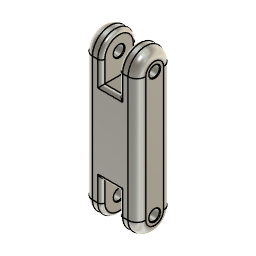
hand_montage v0 (Autodesk Fusion 360 archive; units mm, degrees)
design "proximal v1"
Autodesk Fusion 360 part; units mm, degrees
sketch "Çizim1" plane through (0, 0, 0) normal (0, 1, 0) x (1, 0, 0)
  line L0 (-15, 45) -> (15, 45)
  line L1 (15, 45) -> (15, -45)
  line L2 (15, -45) -> (-15, -45)
  line L3 (-15, -45) -> (-15, 45)
  line L4 (-15, 45) -> (15, -45) construction
  line L5 (15, 45) -> (-15, -45) construction
  dimension "d1" = 30
  dimension "d2" = 90
  constraint horizontal L0
  constraint perpendicular L0 L1
  constraint parallel L0 L2
  constraint parallel L1 L3
  constraint coincident L4 origin
  constraint coincident L5 origin
  measures "d1" distance of L1.end L2.end
  measures "d2" distance of L0.end L1.end
extrude "Ekstrüzyon1" add sketch "Çizim1" along normal blind 20
sketch "Çizim2" plane through (0, 0, 0) normal (0, -1, 0) x (1, 0, 0)
  line L0 (15, 45) -> (-15, 45)
  line L1 (-15, 45) -> (-15, -45)
  line L2 (-15, -45) -> (15, -45)
  line L3 (15, -45) -> (15, 45)
  line L4 (-5, 67) -> (5, 67)
  line L5 (5, 67) -> (5, 23)
  line L6 (5, 23) -> (-5, 23)
  line L7 (-5, 23) -> (-5, 67)
  line L8 (-5, 67) -> (5, 23) construction
  line L9 (5, 67) -> (-5, 23) construction
  point P0 (0, 45)
  dimension "d5" = 10
  dimension "d6" = 44
  constraint horizontal L4
  constraint perpendicular L4 L5
  constraint parallel L4 L6
  constraint parallel L5 L7
  constraint coincident L8 P0
  constraint coincident L9 P0
  constraint midpoint L0 P0
  measures "d5" distance of L5.end L6.end
  measures "d6" distance of L4.end L5.end
extrude "Ekstrüzyon2" cut sketch "Çizim2" against normal blind 70 contours L0 L5 L6 L7
sketch "Çizim3" plane through (0, 0, 0) normal (0, -1, 0) x (1, 0, 0)
  line L0 (-5, 23) -> (-5, 45)
  line L1 (-5, 45) -> (-15, 45)
  line L2 (-15, 45) -> (-15, -45)
  line L3 (-15, -45) -> (15, -45)
  line L4 (15, -45) -> (15, 45)
  line L5 (15, 45) -> (5, 45)
  line L6 (5, 45) -> (5, 23)
  line L7 (5, 23) -> (-5, 23)
  line L8 (-5, -23) -> (5, -23)
  line L9 (5, -23) -> (5, -67)
  line L10 (5, -67) -> (-5, -67)
  line L11 (-5, -67) -> (-5, -23)
  line L12 (-5, -23) -> (5, -67) construction
  line L13 (5, -23) -> (-5, -67) construction
  point P0 (0, -45)
  dimension "d9" = 10
  dimension "d10" = 44
  constraint horizontal L8
  constraint perpendicular L8 L9
  constraint parallel L8 L10
  constraint parallel L9 L11
  constraint coincident L12 P0
  constraint coincident L13 P0
  constraint midpoint L3 P0
  measures "d9" distance of L9.end L10.end
  measures "d10" distance of L8.end L9.end
extrude "Ekstrüzyon3" cut sketch "Çizim3" against normal blind 210 contours L3 L8 L9 L11
sketch "Çizim4" plane through (15, 0, 0) normal (1, 0, 0) x (0, 1, 0)
  line L0 (0, 45) -> (0, -45)
  line L1 (0, -45) -> (20, -45)
  line L2 (20, -45) -> (20, 45)
  line L3 (20, 45) -> (0, 45)
  circle A0 centre (10, 35) radius 10
  circle A1 centre (10, -35) radius 10
  circle A2 centre (10, 35) radius 3
  circle A3 centre (10, -35) radius 3
  dimension "d13" = 20
  dimension "d14" = 20
  dimension "d15" = 6
  dimension "d16" = 6
  constraint concentric A0 A2
  constraint concentric A1 A3
  measures "d13" diameter of A0
  measures "d14" diameter of A1
  measures "d15" diameter of A2
  measures "d16" diameter of A3
extrude "Ekstrüzyon4" cut sketch "Çizim4" against normal blind 52 contours A2 | A3
extrude "Ekstrüzyon5" cut sketch "Çizim4" against normal blind 115 contours L0 L3 A0 | L2 L3 A0 | L0 L1 A1 | L1 L2 A1
fillet "Radyus1" radius 2 16 edges at (-5, 20, 29) (-5, 10, 45) (-5, 0, 29) (5, 0, 29) (5, 10, 45) (5, 20, 29) (5, 0, -29) (5, 10, -45) (5, 20, -29) (-5, 20, -29) (-5, 10, -45) (-5, 0, -29) (0, 0, -23) (0, 0, 23) (0, 20, 23) (0, 20, -23)
fillet "Radyus2" radius 5 8 edges at (15, 10, 45) (15, 20, 0) (15, 10, -45) (15, 0, 0) (-15, 10, -45) (-15, 20, 0) (-15, 10, 45) (-15, 0, 0)
fillet "Radyus3" radius 0.3 8 edges at (-5, 7.203, 36.0848) (-15, 7.203, 33.9152) (5, 7.203, 33.9152) (15, 7.203, 36.0848) (15, 7.203, -33.9152) (5, 7.203, -36.0848) (-5, 7.203, -33.9152) (-15, 7.203, -36.0848)

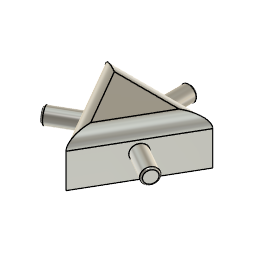
design "wrist_integrator"
Autodesk Fusion 360 part; units mm, degrees
sketch "Çizim5" plane through (0, 0, 0) normal (0, 0, 1) x (1, 0, 0)
  line L0 (-34.641, 20) -> (0, -40)
  line L1 (0, -40) -> (34.641, 20)
  line L2 (34.641, 20) -> (-34.641, 20)
  dimension "d17" = 20
  measures "d17" distance of origin L2
extrude "Ekstrüzyon5" add sketch "Çizim5" along normal blind 30
sketch "Çizim6" plane through (17.3205, -10, 0) normal (0.866025, -0.5, 0) x (0.5, 0.866025, 0)
  line L0 (-34.641, 0) -> (34.641, 0)
  line L1 (34.641, 0) -> (34.641, 30)
  line L2 (34.641, 30) -> (-34.641, 30)
  line L3 (-34.641, 30) -> (-34.641, 0)
  circle A0 centre (0, 15) radius 5
  dimension "d20" = 10
  measures "d20" diameter of A0
extrude "Ekstrüzyon6" add sketch "Çizim6" along normal blind 20 contours A0
sketch "Çizim7" plane through (0, 20, 0) normal (0, 1, 0) x (-1, 0, 0)
  line L0 (-34.641, 0) -> (34.641, 0)
  line L1 (34.641, 0) -> (34.641, 30)
  line L2 (34.641, 30) -> (-34.641, 30)
  line L3 (-34.641, 30) -> (-34.641, 0)
  circle A0 centre (0, 15) radius 5
  dimension "d23" = 10
  measures "d23" diameter of A0
extrude "Ekstrüzyon7" add sketch "Çizim7" along normal blind 20 contours A0
sketch "Çizim8" plane through (-17.3205, -10, 0) normal (-0.866025, -0.5, 0) x (0.5, -0.866025, 0)
  line L0 (-34.641, 0) -> (34.641, 0)
  line L1 (34.641, 0) -> (34.641, 30)
  line L2 (34.641, 30) -> (-34.641, 30)
  line L3 (-34.641, 30) -> (-34.641, 0)
  circle A0 centre (0, 15) radius 5
  dimension "d26" = 10
  measures "d26" diameter of A0
extrude "Ekstrüzyon8" add sketch "Çizim8" along normal blind 20 contours A0
fillet "Radyus3" radius 8 3 edges at (-17.3205, -10, 30) (0, 20, 30) (17.3205, -10, 30)
fillet "Radyus4" radius 1 3 edges at (32.3102, -24.0371, 13.1919) (4.6616, 40, 13.1919) (-36.9718, -15.9629, 13.1919)

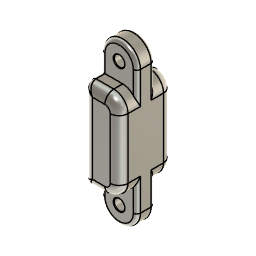
design "middle v1"
Autodesk Fusion 360 part; units mm, degrees
sketch "Çizim1" plane through (0, 0, 0) normal (0, 1, 0) x (1, 0, 0)
  circle A0 centre (0, 0) radius 10
  dimension "d1" = 20
  constraint coincident A0.centre origin
  measures "d1" diameter of A0
extrude "Ekstrüzyon1" add sketch "Çizim1" along normal blind 10
sketch "Çizim2" plane through (0, 0, 0) normal (0, -1, 0) x (1, 0, 0)
  circle A0 centre (0, 0) radius 10
  line L0 (-10, 0) -> (10, 0)
  line L1 (10, 0) -> (10, -80)
  line L2 (10, -80) -> (-10, -80)
  line L3 (-10, -80) -> (-10, 0)
  dimension "d4" = 80
  constraint horizontal L0
  constraint vertical L1
  constraint horizontal L2
  constraint vertical L3
  constraint coincident A0 L0.start
  measures "d4" distance of L0.start L2.end
extrude "Ekstrüzyon2" add sketch "Çizim2" against normal blind 10 contours A0 L1 L2 L3
sketch "Çizim3" plane through (0, 0, 0) normal (0, -1, 0) x (1, 0, 0)
  arc A0 (10, 0) -> (-10, 0) centre (0, 0) ccw
  line L0 (-10, 0) -> (-10, -80)
  line L1 (-10, -80) -> (10, -80)
  line L2 (10, -80) -> (10, 0)
  line L3 (-10, -10) -> (10, -10)
  line L4 (10, -10) -> (10, -60)
  line L5 (10, -60) -> (-10, -60)
  line L6 (-10, -60) -> (-10, -10)
  dimension "d7" = 20
  dimension "d8" = 50
  constraint horizontal L3
  constraint vertical L4
  constraint horizontal L5
  constraint vertical L6
  constraint coincident L0 L3.start
  measures "d7" distance of L3.start L3.end
  measures "d8" distance of L3.start L5.end
extrude "Ekstrüzyon3" add sketch "Çizim3" along normal blind 10 contours L0 L2 L3 L4 L5 L6
sketch "Çizim4" plane through (0, 10, 0) normal (0, 1, 0) x (-1, 0, 0)
  arc A0 (10, 0) -> (-10, 0) centre (0, 0) ccw
  line L0 (-10, 0) -> (-10, -80)
  line L1 (-10, -80) -> (10, -80)
  line L2 (10, -80) -> (10, 0)
  line L3 (-10, -10) -> (10, -10)
  line L4 (10, -10) -> (10, -60)
  line L5 (10, -60) -> (-10, -60)
  line L6 (-10, -60) -> (-10, -10)
  dimension "d11" = 50
  constraint horizontal L3
  constraint vertical L4
  constraint horizontal L5
  constraint vertical L6
  constraint coincident L0 L3.start
  measures "d11" distance of L3.start L5.end
extrude "Ekstrüzyon4" add sketch "Çizim4" along normal blind 10 contours L0 L2 L3 L4 L5 L6
sketch "Çizim5" plane through (0, 0, 0) normal (0, -1, 0) x (1, 0, 0)
  line L0 (10, -60) -> (-10, -60)
  line L1 (-10, -60) -> (-10, -80)
  line L2 (-10, -80) -> (10, -80)
  line L3 (10, -80) -> (10, -60)
  circle A0 centre (0, -70) radius 10
  dimension "d14" = 20
  measures "d14" diameter of A0
extrude "Ekstrüzyon5" cut sketch "Çizim5" against normal blind 15 contours L2 L3 A0 | L1 L2 A0
sketch "Çizim6" plane through (0, 10, 0) normal (0, 1, 0) x (-1, 0, 0)
  line L0 (-10, -10) -> (10, -10)
  line L1 (10, -10) -> (10, 0)
  arc A0 (10, 0) -> (-10, 0) centre (0, 0) ccw
  line L2 (-10, 0) -> (-10, -10)
  circle A1 centre (0, 0) radius 3
  dimension "d17" = 6
  constraint coincident A0.centre A1.centre
  measures "d17" diameter of A1
extrude "Ekstrüzyon6" cut sketch "Çizim6" against normal blind 105 contours A1
sketch "Çizim7" plane through (0, 10, 0) normal (0, 1, 0) x (-1, 0, 0)
  arc A0 (-10, -70) -> (10, -70) centre (0, -70) ccw
  line L0 (10, -70) -> (10, -60)
  line L1 (10, -60) -> (-10, -60)
  line L2 (-10, -60) -> (-10, -70)
  circle A1 centre (0, -70) radius 3
  dimension "d20" = 6
  constraint concentric A0 A1
  measures "d20" diameter of A1
extrude "Ekstrüzyon7" cut sketch "Çizim7" against normal blind 34 contours A1
fillet "Radyus1" radius 2 12 edges at (-10, 0, -5) (0, 0, 10) (10, 0, -5) (-10, 10, -5) (0, 10, 10) (10, 10, -5) (10, 0, -65) (0, 0, -80) (-10, 0, -65) (10, 10, -65) (0, 10, -80) (-10, 10, -65)
fillet "Radyus2" radius 5 2 faces at (-3.3333, -10, -43.3333) (3.3333, 20, -43.3333)
fillet "Radyus3" radius 0.3 4 edges at (2.797, 0, -1.0848) (2.797, 10, 1.0848) (2.797, 0, -71.0848) (2.797, 10, -68.9152)
fillet "Radyus4" radius 8 8 edges at (10, -1.5, -10) (8.5355, -8.5355, -11.4645) (10, 11.5, -10) (8.5355, 18.5355, -11.4645) (10, -1.5, -60) (8.5355, -8.5355, -58.5355) (10, 11.5, -60) (8.5355, 18.5355, -58.5355)
fillet "Radyus5" radius 2 8 edges at (-10, 11.5, -10) (-8.5355, 18.5355, -11.4645) (-10, -1.5, -10) (-8.5355, -8.5355, -11.4645) (-10, 11.5, -60) (-8.5355, 18.5355, -58.5355) (-10, -1.5, -60) (-8.5355, -8.5355, -58.5355)

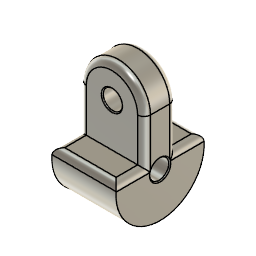
design "knuckle"
Autodesk Fusion 360 part; units mm, degrees
sketch "Çizim1" plane through (0, 0, 0) normal (0, 1, 0) x (1, 0, 0)
  circle A0 centre (0, 0) radius 10
  dimension "d1" = 20
  constraint coincident A0.centre origin
  measures "d1" diameter of A0
extrude "Ekstrüzyon1" add sketch "Çizim1" along normal blind 10
sketch "Çizim2" plane through (0, 0, 0) normal (0, -1, 0) x (1, 0, 0)
  circle A0 centre (0, 0) radius 10
  line L0 (-10, 0) -> (10, 0)
  line L1 (10, 0) -> (10, -30)
  line L2 (10, -30) -> (-10, -30)
  line L3 (-10, -30) -> (-10, 0)
  dimension "d4" = 30
  constraint horizontal L0
  constraint vertical L1
  constraint horizontal L2
  constraint vertical L3
  constraint coincident A0 L0.start
  measures "d4" distance of L0.start L2.end
extrude "Ekstrüzyon2" add sketch "Çizim2" against normal blind 10 contours A0 L1 L2 L3
sketch "Çizim3" plane through (10, 0, 0) normal (1, 0, 0) x (0, 1, 0)
  line L0 (0, 0) -> (0, -30)
  line L1 (0, -30) -> (10, -30)
  line L2 (10, -30) -> (10, 0)
  line L3 (10, 0) -> (0, 0)
  circle A0 centre (5, -16.25) radius 13.75
  dimension "d7" = 27.5
  measures "d7" diameter of A0
extrude "Ekstrüzyon3" add sketch "Çizim3" against normal blind 20 contours L0 A0 | L2 A0
sketch "Çizim4" plane through (10, 0, 0) normal (1, 0, 0) x (0, 1, 0)
  line L0 (0, 0) -> (0, -3.4413)
  arc A0 (0, -3.4413) -> (0, -29.0587) centre (5, -16.25) ccw
  line L1 (0, -29.0587) -> (0, -30)
  line L2 (0, -30) -> (10, -30)
  line L3 (10, -30) -> (10, -29.0587)
  arc A1 (10, -29.0587) -> (10, -3.4413) centre (5, -16.25) ccw
  line L4 (10, -3.4413) -> (10, 0)
  line L5 (10, 0) -> (0, 0)
  circle A2 centre (5, -16.25) radius 13.75
  constraint tangent A1 A2
extrude "Ekstrüzyon4" cut sketch "Çizim4" against normal blind 35 contours L1 L2 A2 | L2 L3 A2
sketch "Çizim5" plane through (0, 0, 0) normal (0, -1, 0) x (1, 0, 0)
  line L0 (-10, -3.4413) -> (10, -3.4413)
  line L1 (10, -3.4413) -> (10, 0)
  arc A0 (10, 0) -> (-10, 0) centre (0, 0) ccw
  line L2 (-10, 0) -> (-10, -3.4413)
  circle A1 centre (0, 0) radius 3
  dimension "d12" = 6
  constraint coincident A0.centre A1.centre
  measures "d12" diameter of A1
extrude "Ekstrüzyon5" cut sketch "Çizim5" against normal blind 80 contours A1
sketch "Çizim6" plane through (10, 0, 0) normal (1, 0, 0) x (0, 1, 0)
  arc A0 (0, -3.4413) -> (10, -3.4413) centre (5, -16.25) ccw
  line L0 (10, -3.4413) -> (10, 0)
  line L1 (10, 0) -> (0, 0)
  line L2 (0, 0) -> (0, -3.4413)
  line L3 (0, -3.4413) -> (10, -3.4413)
  line L4 (10, -3.4413) -> (10, -13.4413)
  line L5 (10, -13.4413) -> (0, -13.4413)
  line L6 (0, -13.4413) -> (0, -3.4413)
  line L7 (-8.4601, -13.4413) -> (18.4601, -13.4413)
  dimension "d15" = 10
  constraint horizontal L3
  constraint vertical L4
  constraint horizontal L5
  constraint vertical L6
  constraint coincident A0.start L2.end
  constraint coincident A0 L7.start
  constraint coincident A0 L7.end
  constraint perpendicular L6 L7
  measures "d15" distance of A0.start L5.end
extrude "Ekstrüzyon6" cut sketch "Çizim6" against normal blind 39 contours A0 L6 L7 | A0 L4 L7
fillet "Radyus1" radius 2 6 edges at (0, 18.4601, -13.4413) (0, -8.4601, -13.4413) (10, -4.23, -13.4413) (10, 14.23, -13.4413) (-10, -4.23, -13.4413) (-10, 14.23, -13.4413)
fillet "Radyus2" radius 2 6 edges at (-10, 10, -7.7207) (0, 10, 10) (10, 10, -7.7207) (-10, 0, -7.7207) (0, 0, 10) (10, 0, -7.7207)
fillet "Radyus3" radius 0.3 1 edges at (-2.797, 10, -1.0848)
sketch "Çizim7" plane through (10, 0, 0) normal (1, 0, 0) x (0, 1, 0)
  line L0 (2, -15.4413) -> (-8.7262, -15.4413)
  arc A0 (-8.7262, -15.4413) -> (18.7262, -15.4413) centre (5, -16.25) ccw
  line L1 (18.7262, -15.4413) -> (8, -15.4413)
  line L2 (8, -15.4413) -> (8, 0)
  line L3 (8, 0) -> (2, 0)
  line L4 (2, 0) -> (2, -15.4413)
  circle A1 centre (5, -16.25) radius 13.75
  circle A2 centre (5, -16.25) radius 3
  dimension "d24" = 27.5
  dimension "d25" = 6
  constraint concentric A1 A2
  measures "d24" diameter of A1
  measures "d25" diameter of A2
extrude "Ekstrüzyon7" cut sketch "Çizim7" against normal blind 30 contours A2
fillet "Radyus4" radius 0.3 3 edges at (10, 2.203, -15.1652) (-10, 2.203, -17.3348) (-2.797, 0, 1.0848)
